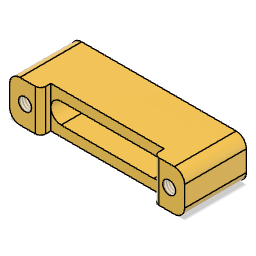
soporte_arduino_back_v6 (Autodesk Fusion 360 design; units mm, degrees)
Autodesk Fusion 360 part; units mm, degrees
sketch "Sketch1" plane through (0, 0, 0) normal (0, 0, 1) x (1, 0, 0)
  line L0 (17, 4) -> (-17, 4)
  line L1 (-17, 4) -> (-17, -4)
  line L2 (-17, -4) -> (17, -4)
  line L3 (17, -4) -> (17, 4)
  line L4 (17, 4) -> (-17, -4) construction
  line L5 (-17, 4) -> (17, -4) construction
  line L6 (0, 0) -> (14, 0) construction
  circle A0 centre (14, 0) radius 1.5
  line L7 (0, 0) -> (0, 4) construction
  circle A1 centre (-14, 0) radius 1.5
  line L8 (11, 2) -> (-11, 2)
  line L9 (-11, 2) -> (-11, -2)
  line L10 (-11, -2) -> (11, -2)
  line L11 (11, -2) -> (11, 2)
  line L12 (11, 2) -> (-11, -2) construction
  line L13 (-11, 2) -> (11, -2) construction
  line L14 (-11, -4) -> (11, -4)
  line L15 (11, -4) -> (11, 4)
  line L16 (11, 4) -> (-11, 4)
  line L17 (-11, 4) -> (-11, -4)
  line L18 (-11, -4) -> (11, 4) construction
  line L19 (11, -4) -> (-11, 4) construction
  dimension "d44" = 34
  dimension "d45" = 14
  dimension "d46" = 3
  dimension "d47" = 3
  dimension "d48" = 2
  dimension "d49" = 8
  dimension "d54" = 22
  constraint horizontal L0
  constraint perpendicular L0 L1
  constraint parallel L0 L2
  constraint parallel L1 L3
  constraint coincident L4 L6.start
  constraint coincident L5 L6.start
  constraint coincident L6.start L7.start
  constraint horizontal L6
  constraint coincident L6.end A0.centre
  constraint midpoint L0 L7.end
  constraint symmetric A0 L7 A1
  constraint horizontal L8
  constraint perpendicular L8 L9
  constraint parallel L8 L10
  constraint parallel L9 L11
  constraint coincident L12 L6.start
  constraint coincident L13 L6.start
  constraint horizontal L14
  constraint perpendicular L14 L15
  constraint parallel L14 L16
  constraint parallel L15 L17
  constraint coincident L18 L6.start
  constraint coincident L19 L6.start
  constraint coincident L2 L14.start
  measures "d44" distance of L1.end L2.end
  measures "d45" distance of L6.start L6.end
  measures "d46" diameter of A0
  measures "d47" distance of L6.end L11
  measures "d48" distance of L2 L10
  measures "d49" distance of L0.start L2.end
  measures "d54" distance of L15 L17
extrude "Extrude4" add sketch "Sketch1" against normal blind 12 contours L0 L2 L3 L11 L15 | L0 L8 L15 L16 L17 | L0 L1 L2 L9 L17 | L2 L10 L14 L15 L17
fillet "Fillet5" radius 2 8 edges at (-17, -4, -6) (17, -4, -6) (17, 4, -6) (-17, 4, -6) (-11, 2, -6) (-11, -2, -6) (11, -2, -6) (11, 2, -6)
thread "Thread4" "ISO Metric profile 3.0 M3x0.5 6H" major diameter 3.086 minor diameter 2.529 pitch 0.5 angle 60 resizes the face on face at (15.4981, -0.0748, -8) on face at (-12.5019, -0.0748, -8)
extrude "Extrude5" cut sketch "Sketch1" against normal blind 2 contours L0 L8 L15 L16 L17 | L8 L9 L10 L11 L15 L17 | L2 L10 L14 L15 L17
fillet "Fillet6" radius 1 2 edges at (-11, 0, 0) (11, 0, 0)
equation "d1 = ( 47 / 2 ) * 1 mm"
